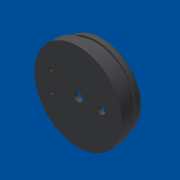
# Autodesk Inventor part: Deckel_oben
Saved by Autodesk Inventor 2018.3 (Build 223284000, 284)
## iProperties
Created: 2016-11-15
Part Number: Deckel_oben
Material: PVC, hart
Document SubType Name: Modeling
Designer: stud_brinkmann
Mass: 48.9925 g
Surface Area: 143.372 cm^2
Volume: 37.9787 cm^3
Density: 1.29 g/cm^3
Appearance: Glatt - weiß
Author: stud_brinkmann
Autodesk Inventor part; units mm, degrees
ref_plane "YZ Plane" through (0, 0, 0) normal (1, 0, 0) x (0, 1, 0)
ref_plane "XZ Plane" through (0, 0, 0) normal (0, 1, 0) x (-1, 0, 0)
ref_plane "XY Plane" through (0, 0, 0) normal (0, 0, 1) x (1, 0, 0)
sketch "Skizze2" plane through (0, 0, 0) normal (1, 0, 0) x (0, 1, 0)
  line L0 (0, 0) -> (18.8, 0)
  line L1 (0, 3.1) -> (3, 3.1)
  line L2 (18.8, 31.354) -> (17.3, 31.9)
  line L3 (17.3, 31.9) -> (14.3, 31.9)
  line L4 (14.3, 31.9) -> (14.3, 30.15)
  line L5 (14.3, 30.15) -> (10.8, 30.15)
  line L6 (10.8, 30.15) -> (10.8, 31.9)
  line L7 (10.8, 31.9) -> (7.8, 31.9)
  line L8 (7.8, 31.9) -> (7.8, 35)
  line L9 (7.8, 35) -> (0, 35)
  line L10 (18.8, 31.354) -> (18.8, 27)
  line L11 (18.8, 27) -> (3, 27)
  line L12 (3, 27) -> (3, 3.1)
  line L13 (0, 35) -> (0, 3.1)
  dimension "d5" = 6.2
  dimension "d10" = 20
  dimension "d11" = 60.3
  dimension "d12" = 63.8
  dimension "d26" = 70
  dimension "d34" = 1.5
  dimension "d35" = 4.5
  dimension "d36" = 8
  dimension "d37" = 11
  dimension "d39" = 3
  dimension "d41" = 18.8
  dimension "d50" = 54
  constraints: 28 end point, 7 perpendicular, 2 horizontal, 2 point on line, 2 vertical, 2 vertical alignment, 1 parallel, 1 other
  measures "d5" diameter of L1 L0
  measures "d10" angle of L3 L2
  measures "d11" diameter of L5 L0
  measures "d12" diameter of L3 L0
  measures "d26" diameter of L9 L0
  measures "d34" distance from line of L2.end L10
  measures "d35" distance between parallel lines of L4 L10
  measures "d36" distance between parallel lines of L6 L10
  measures "d37" distance between parallel lines of L8 L10
  measures "d39" distance of L1.start L1.end
  measures "d41" distance between parallel lines of L13 L10
  measures "d50" diameter of L11 L0
revolve "Umdrehung1" add sketch "Skizze2" angle 360 about axis through (0, 0, 0) along (0, 1, 0)
fillet "Rundung1" radius 0.4 2 edges at (0, 10.8, -30.15) (0, 14.3, -30.15)
chamfer "Fase1" distance 0.5 angle 45 1 edges at (0, 0, -3.1)
sketch "Skizze7" plane through (0, 3, 0) normal (0, 1, 0) x (1, 0, 0)
  arc A0 (-7.5, -18.4326) -> (7.5, -18.4326) centre (0, 0) ccw
  circle A1 centre (0, 0) radius 31.9 projected
  line L0 (0, 49) -> (0, -49) projected
  line L1 (-7.5, -18.4326) -> (-7.5, -25.9374)
  circle A2 centre (0, 0) radius 27 projected
  line L2 (7.5, -18.4326) -> (7.5, -25.9374)
  arc A3 (-7.5, -25.9374) -> (7.5, -25.9374) centre (0, 0) ccw
  line L3 (7.5, 18.4326) -> (7.5, 25.9374)
  arc A4 (7.5, 18.4326) -> (-7.5, 18.4326) centre (0, 0) ccw
  arc A5 (7.5, 25.9374) -> (-7.5, 25.9374) centre (0, 0) ccw
  line L4 (-7.5, 18.4326) -> (-7.5, 25.9374)
  dimension "d70" = 12
  dimension "d73" = 360
  dimension "d75" = 15
  constraints: 10 point on circle, 8 end point, 4 centre point, 1 coincident, 1 concentric, 1 parallel, 22 other
  measures "d70" radial gap between concentric circles of A1 A0
  measures "d75" distance between parallel lines of L2 L1
extrude "Extrusion2" add sketch "Skizze7" along normal blind 10 contours A0 L0 A2 L1 | A0 L2 A2 L0 | A4 L4 A2 L0 | L0 A2 L3 A4
sketch "Skizze8" plane through (0, 13, 0) normal (0, 1, 0) x (1, 0, 0)
  line L0 (0, 49) -> (0, -49) projected
  point P0 (0, 0)
  point P1 (0, -23.5)
  dimension "d78" = 23.5
  constraints: 1 point on line
  measures "d78" distance of point (0, 0) point (0, -23.5)
hole "Bohrung3" at (0, 13, 23.5) direction (0, -1, 0) diameter 2.5 depth 8 tip angle 118
thread "Gewinde1" size "M3x0.5" class "6H" standard "ANSI Metric M Profile" full length
pattern_circular "Runde Anordnung1" count 2 over 360 about axis through (0, 10.9, 0) along (0, 1, 0) of "Bohrung3"
sketch "Skizze9" plane through (0, 0, 0) normal (0, -1, 0) x (1, 0, 0)
  line L0 (-49, 0) -> (49, 0) projected
  point P0 (0, 0)
  point P1 (-22, -8)
  point P2 (-22, 8)
  dimension "d91" = 16
  dimension "d92" = 22
  constraints: 1 symmetric about line
  measures "d91" distance of point (-22, 8) point (-22, -8)
  measures "d92" horizontal distance of point (-22, 8) point (0, 0)
hole "Bohrung4" at (-22, 0, -8) at (-22, 0, 8) direction (0, 1, 0) diameter 3.3 end through all
thread "Gewinde2" size "M4x0.7" class "6H" standard "ANSI Metric M Profile" full length
thread "Gewinde3" size "M4x0.7" class "6H" standard "ANSI Metric M Profile" full length
sketch "Skizze10" plane through (0, 13, 0) normal (0, 1, 0) x (1, 0, 0)
  point P0 (0, 0)
  point P1 (4, -23.5)
  dimension "d104" = 23.5
  dimension "d105" = 4
  measures "d104" vertical distance of point (4, -23.5) point (0, 0)
  measures "d105" horizontal distance of point (0, 0) point (4, -23.5)
hole "Bohrung5" at (4, 13, 23.5) direction (0, -1, 0) diameter 0.8 end through all
hole "Bohrung6" at (4, 0, 23.5) direction (0, 1, 0) diameter 1.6 depth 5 tip angle 118
thread "Gewinde4" size "M2x0.4" class "6H" standard "ANSI Metric M Profile" full length
sketch "Skizze11" plane through (0, 3, 0) normal (0, 1, 0) x (1, 0, 0)
  line L0 (-49, 0) -> (49, 0) projected
  point P0 (0, 0)
  point P1 (18.4, 0)
  dimension "d124" = 18.4
  constraints: 1 point on line
  measures "d124" distance of point (0, 0) point (18.4, 0)
hole "Bohrung7" at (18.4, 3, 0) direction (0, -1, 0) diameter 6 end through all
fillet "Rundung2" radius 2 4 edges at (7.5, 8, 25.9374) (-7.5, 8, 25.9374) (7.5, 8, -25.9374) (-7.5, 8, -25.9374)
equation "\"d36\" = d35 + ORing1"
equation "\"ORing1\" = 3.5"
